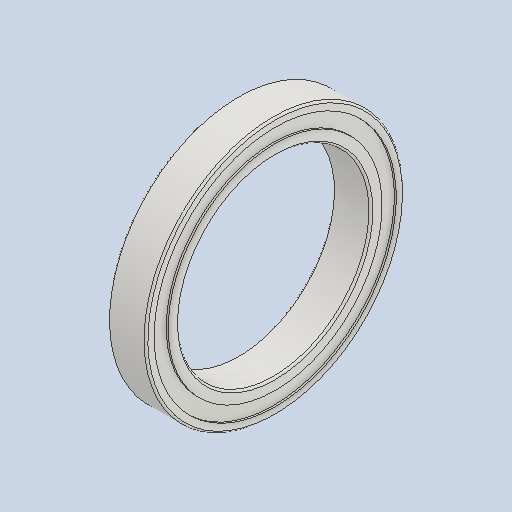
# Autodesk Inventor part: C-E6704ZZ
Saved by Autodesk Inventor 2025.3 (Build 293356030, 356C)
## iProperties
Category: PARTsolutions
Company: MISUMI
Created: 2025-09-20
Part Number: C-E6704ZZ
Material: 강철, 가공됨
Catalog Web Link: www.cadenas.de
Description: C-E6___ZZ-Economy Deep Groove Ball Bearing - Double Shielded, Single Row
Vendor: MISUMI
Document SubType Name: Modeling
Designer: psAdmin
Manufacturer: MISUMI
Mass: 7.74818 g
Surface Area: 11.4195 cm^2
Volume: 0.987029 cm^3
Density: 7.85 g/cm^3
Appearance: 강철
PSOL_IDENT_0: {$CADENAS_DATA/23d-libs/misumi/metric/12_bearing_holders/c_e6700zz.prj},162 {VTYP=3D},{NB=C-E6704ZZ}
PSOL_IDENT_1: ,{LINA=C-E6704ZZ},{NN=C-E6___ZZ},{DATE=29.05.2023 02:13:12},{GEOMDATE=25.05.2021 01:16:58},{VERSION=
PSOL_IDENT_2: },{LINEID=620},{WBVAR=},{WBNUMERIC=}  {NB=C-E6704ZZ},{LINA=C-E6704ZZ},{KT=DUMMY},{PN=C-E6704ZZ},{TS=
PSOL_IDENT_3: C-E6704ZZ},{DD=20},{D=27},{B=4},{RR=0.2},{AA=3.6000},{BB=0.8500},{CC=1.1800}
NB: C-E6704ZZ
NN: C-E6___ZZ
NT: Economy Deep Groove Ball Bearing - Double Shielded, Single Row
NBSYN: $PN.
LINA: C-E6704ZZ
CATALOG: Misumi
PN: C-E6704ZZ
TS: C-E6704ZZ
DD: 20
D: 27
B: 4
RR: 0.2
SUPPLIER: MISUMI
ARTICLENO: C-E6704ZZ
BOMINFO: C-E6704ZZ
CREATOR: CADENAS GmbH
Title: C-E6704ZZ
Author: Cadenas PARTsolutions
Comments: Economy Deep Groove Ball Bearing - Double Shielded, Single Row
Autodesk Inventor part; units mm, degrees
sketch "Sketch_1" plane through (0, 0, 0) normal (0, 0, 1) x (1, 0, 0)
  line L0 (4, 0) -> (0, 0)
  arc A0 (0, 10.2) -> (0.2, 10) centre (0.2, 10.2) ccw
  line L1 (0.2, 10) -> (3.8, 10)
  arc A1 (3.8, 10) -> (4, 10.2) centre (3.8, 10.2) ccw
  line L2 (4, 10.2) -> (4, 11.18)
  line L3 (4, 11.18) -> (3.8, 11.18)
  line L4 (3.8, 11.18) -> (3.8, 12.65)
  line L5 (3.8, 12.65) -> (4, 12.65)
  line L6 (4, 12.65) -> (4, 13.3)
  arc A2 (4, 13.3) -> (3.8, 13.5) centre (3.8, 13.3) ccw
  line L7 (3.8, 13.5) -> (0.2, 13.5)
  arc A3 (0.2, 13.5) -> (0, 13.3) centre (0.2, 13.3) ccw
  line L8 (0, 13.3) -> (0, 12.65)
  line L9 (0, 12.65) -> (0.2, 12.65)
  line L10 (0.2, 12.65) -> (0.2, 11.18)
  line L11 (0.2, 11.18) -> (0, 11.18)
  line L12 (0, 11.18) -> (0, 10.2)
  constraints: 26 end point, 8 point on circle, 4 centre point
revolve "Revolution1" add sketch "Sketch_1" angle 360 about axis through (4, 0, 0) along (1, 0, 0)
ref_plane "center_point_XY" through (2, 0, 0) normal (1, 0, 0) x (0, 0, -1)
ref_plane "center_point_YZ" through (2, 0, 0) normal (0, 0, -1) x (0, 1, 0)
ref_plane "center_point_ZX" through (2, 0, 0) normal (0, 1, 0) x (1, 0, 0)
ref_plane "to_housing_XY" through (0, 0, 0) normal (1, 0, 0) x (0, 0, -1)
ref_plane "to_housing_YZ" through (0, 0, 0) normal (0, 0, -1) x (0, 1, 0)
ref_plane "to_housing_ZX" through (0, 0, 0) normal (0, 1, 0) x (1, 0, 0)
ref_plane "to_ring_XY" through (3.6, 0, 0) normal (1, 0, 0) x (0, 0, -1)
ref_plane "to_ring_YZ" through (3.6, 0, 0) normal (0, 0, -1) x (0, 1, 0)
ref_plane "to_ring_ZX" through (3.6, 0, 0) normal (0, 1, 0) x (1, 0, 0)
body "Solid1"
